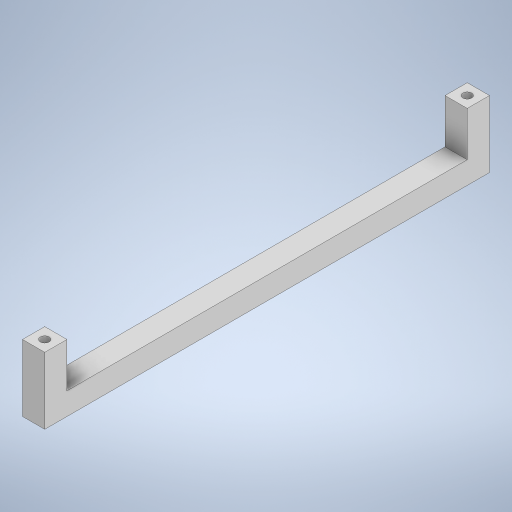
# Autodesk Inventor part: handle ds
Saved by Autodesk Inventor 2023 (Build 270158000, 158)
## iProperties
Created: 2023-12-23
Part Number: handle ds
Material: Generic
Document SubType Name: Modeling
Designer: elija
Density: 1 g/cm^3
Appearance: Default
Author: elija
Autodesk Inventor part; units mm, degrees
ref_plane "YZ Plane" through (0, 0, 0) normal (1, 0, 0) x (0, 1, 0)
ref_plane "XZ Plane" through (0, 0, 0) normal (0, 1, 0) x (-1, 0, 0)
ref_plane "XY Plane" through (0, 0, 0) normal (0, 0, 1) x (1, 0, 0)
sketch "Sketch1" plane through (0, 0, 0) normal (0, 1, 0) x (-1, 0, 0)
  line L0 (0, 0) -> (-12.7, 0)
  line L1 (-12.7, 0) -> (-12.7, -254)
  line L2 (-12.7, -254) -> (0, -254)
  line L3 (0, -254) -> (0, 0)
  dimension "d0" = 254
  dimension "d1" = 12.7
  constraints: 8 end point, 2 parallel, 1 horizontal, 1 perpendicular
  measures "d0" distance of L2.end L0.start
  measures "d1" distance of L1.end L2.end
extrude "Extrusion1" add sketch "Sketch1" along normal blind 12.7
sketch "Sketch2" plane through (0, 12.7, 0) normal (0, 1, 0) x (1, 0, 0)
  line L0 (12.7, 0) -> (12.7, 254) projected
  line L1 (0, 0) -> (12.7, 0)
  line L2 (12.7, 0) -> (12.7, 12.7)
  line L3 (12.7, 12.7) -> (0, 12.7)
  line L4 (0, 12.7) -> (0, 0)
  line L5 (12.7, 254) -> (0, 254) projected
  line L6 (0, 254) -> (12.7, 254)
  line L7 (12.7, 254) -> (12.7, 241.3)
  line L8 (12.7, 241.3) -> (0, 241.3)
  line L9 (0, 241.3) -> (0, 254)
  dimension "d4" = 12.7
  constraints: 16 end point, 5 parallel, 3 perpendicular, 2 horizontal, 2 point on line
  measures "d4" distance of L8.end L5.end
extrude "Extrusion2" add sketch "Sketch2" along normal blind 25.4
sketch "Sketch3" plane through (0, 38.1, 0) normal (0, 1, 0) x (1, 0, 0)
  circle A0 centre (6.35, 6.35) radius 2.5019
  line L0 (0, 0) -> (12.7, 0) projected
  line L1 (12.7, 0) -> (12.7, 12.7) projected
  circle A1 centre (6.35, 247.65) radius 2.5019
  dimension "d7" = 5.0038
  dimension "d8" = 6.35
  dimension "d9" = 6.35
  dimension "d12" = 241.3
  constraints: 2 centre point, 1 vertical, 2 other
  measures "d7" diameter of A0
  measures "d8" distance from line of L0 A0.centre
  measures "d9" distance from line of L1 A0.centre
  measures "d12" distance of A0.centre A1.centre
extrude "Extrusion3" cut sketch "Sketch3" against normal up to surface (38.1 mm away)
body "Solid1"
